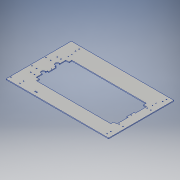
# Autodesk Inventor part: Hopper Top
Saved by Autodesk Inventor 2018 (Build 220112000, 112)
## iProperties
Created: 2013-10-16
Part Number: Hopper Top
Material: Aluminum 6061
Document SubType Name: Modeling
Designer: Gabriel Smolnycki
Mass: 1199.4 g
Surface Area: 2361.58 cm^2
Volume: 444.221 cm^3
Density: 2.7 g/cm^3
Appearance: Aluminum - Flat
Sending System: SolidWorks 2017
Last Author: Gabriel Smolnycki
Last Saved: 2017-09-14
Author: Gabriel Smolnycki
Autodesk Inventor part; units mm, degrees
ref_plane "YZ Plane" through (0, 0, 0) normal (1, 0, 0) x (0, 1, 0)
ref_plane "XY Plane" through (0, 0, 0) normal (0, 0, 1) x (1, 0, 0)
ref_plane "Work Plane1" through (0, -4, 0) normal (0, 1, 0) x (-1, 0, 0)
sketch "Sketch1" plane through (0, -4, 0) normal (0, 1, 0) x (-1, 0, 0)
  line L0 (209, 19.5) -> (209, -19.5)
  line L1 (-216.3969, -79.4609) -> (-199.5, -79.4609)
  line L2 (221, -27.5) -> (216.3969, -27.5)
  line L3 (-209, -19.5) -> (-209, 19.5)
  line L4 (290, 167.5) -> (-260, 167.5)
  line L5 (-199.5, 79.4609) -> (-216.3969, 79.4609)
  line L6 (-260, -182.5) -> (290, -182.5)
  line L7 (199.5, 79.4609) -> (199.5, 95)
  line L8 (221, 47.5) -> (216.3969, 47.5)
  line L9 (216.3969, -79.4609) -> (216.3969, -47.5)
  line L10 (216.3969, 19.5) -> (216.3969, 27.5)
  line L11 (-199.5, -95) -> (199.5, -95)
  line L12 (209, -19.5) -> (216.3969, -19.5)
  line L13 (-216.3969, -19.5) -> (-216.3969, -79.4609)
  arc A0 (221, -47.5) -> (221, -27.5) centre (221, -37.5) ccw
  line L14 (-209, 19.5) -> (-216.3969, 19.5)
  line L15 (-199.5, 95) -> (-199.5, 79.4609)
  line L16 (-260, 167.5) -> (-260, -182.5)
  line L17 (216.3969, 79.4609) -> (199.5, 79.4609)
  arc A1 (221, 27.5) -> (221, 47.5) centre (221, 37.5) ccw
  line L18 (199.5, -79.4609) -> (216.3969, -79.4609)
  line L19 (290, -182.5) -> (290, 167.5)
  line L20 (216.3969, 19.5) -> (209, 19.5)
  line L21 (-199.5, -79.4609) -> (-199.5, -95)
  line L22 (216.3969, -27.5) -> (216.3969, -19.5)
  line L23 (-216.3969, -19.5) -> (-209, -19.5)
  line L24 (216.3969, -47.5) -> (221, -47.5)
  line L25 (-216.3969, 79.4609) -> (-216.3969, 19.5)
  line L26 (199.5, 95) -> (-199.5, 95)
  line L27 (216.3969, 47.5) -> (216.3969, 79.4609)
  line L28 (216.3969, 27.5) -> (221, 27.5)
  line L29 (199.5, -95) -> (199.5, -79.4609)
  point P0 (0, 0)
  dimension "d194" = 79.4609
  dimension "d195" = 216.3969
  dimension "d196" = 216.3969
  dimension "d197" = 79.4609
  dimension "d198" = 209
  dimension "d199" = 19.5
  dimension "d201" = 20
  dimension "d202" = 27.5
  dimension "d203" = 10
  dimension "d204" = 95
  dimension "d205" = 199.5
  dimension "d206" = 260
  dimension "d207" = 550
  dimension "d208" = 182.5
  dimension "d209" = 350
  dimension "d210" = 221
  dimension "d211" = 4.6031
  constraints: 60 end point, 16 horizontal, 14 vertical, 13 equal length, 6 collinear, 4 point on circle, 2 centre point, 1 equal radius, 1 other
  measures "d194" distance from line of L18 point (0, 0)
  measures "d195" distance from line of point (0, 0) L9
  measures "d196" distance from line of L13 point (0, 0)
  measures "d197" distance from line of L17 point (0, 0)
  measures "d198" distance from line of L0 point (0, 0)
  measures "d199" distance from line of L12 point (0, 0)
  measures "d201" distance between parallel lines of L2 L24
  measures "d202" distance from line of L2 point (0, 0)
  measures "d203" radius of A0
  measures "d204" distance from line of point (0, 0) L11
  measures "d205" distance from line of point (0, 0) L29
  measures "d206" distance from line of L16 point (0, 0)
  measures "d207" distance between parallel lines of L19 L16
  measures "d208" distance from line of L6 point (0, 0)
  measures "d209" distance between parallel lines of L4 L6
  measures "d210" horizontal distance of point (0, 0) L2.start
  measures "d211" distance of L9.end L24.end
extrude "Extrusion2" add sketch "Sketch1" along normal blind 4
sketch "Sketch2" plane through (0, 0, 0) normal (0, 1, 0) x (-1, 0, 0)
  arc A0 (144, 149.75) -> (144, 145.25) centre (144, 147.5) ccw
  line L0 (154, 149.75) -> (144, 149.75)
  line L1 (144, 145.25) -> (154, 145.25)
  arc A1 (154, 145.25) -> (154, 149.75) centre (154, 147.5) ccw
  constraints: 4 end point, 4 point on circle, 2 centre point, 2 horizontal, 1 equal radius, 1 parallel
extrude "Extrusion1" cut sketch "Sketch2" against normal blind 4
hole "Hole27" at (-281.5, -4, 37.5) direction (0, 1, 0) diameter 4.5 depth 4
hole "Hole26" at (-256.5, -4, -37.5) direction (0, 1, 0) diameter 4.5 depth 4
hole "Hole25" at (-281.5, -4, -37.5) direction (0, 1, 0) diameter 4.5 depth 4
hole "Hole24" at (214, -4, 0) direction (0, 1, 0) diameter 3.5 depth 4
hole "Hole23" at (-214, -4, 0) direction (0, 1, 0) diameter 3.5 depth 4
hole "Hole22" at (-284, -4, 147.5) direction (0, 1, 0) diameter 4.5 depth 4
hole "Hole21" at (236, -4, 131.5) direction (0, 1, 0) diameter 4.5 depth 4
hole "Hole20" at (236, -4, 151.5) direction (0, 1, 0) diameter 4.5 depth 4
hole "Hole19" at (236, -4, -166.5) direction (0, 1, 0) diameter 4.5 depth 4
hole "Hole18" at (236, -4, -146.5) direction (0, 1, 0) diameter 4.5 depth 4
hole "Hole17" at (-232, -4, 131.5) direction (0, 1, 0) diameter 4.5 depth 4
hole "Hole16" at (-232, -4, 151.5) direction (0, 1, 0) diameter 4.5 depth 4
hole "Hole15" at (-232, -4, -166.5) direction (0, 1, 0) diameter 4.5 depth 4
sketch "Sketch16" plane through (0, -4, 0) normal (0, 1, 0) x (-1, 0, 0)
  point P0 (232, -146.5)
hole "Hole14" at (-232, -4, -146.5) direction (0, 1, 0) diameter 4.5 depth 4
sketch "Sketch15" plane through (0, -4, 0) normal (0, 1, 0) x (-1, 0, 0)
  point P0 (232, -166.5)
hole "Hole13" at (225.5, -4, -121) direction (0, 1, 0) diameter 3.5 depth 4
sketch "Sketch14" plane through (0, -4, 0) normal (0, 1, 0) x (-1, 0, 0)
  point P0 (232, 151.5)
hole "Hole12" at (225.5, -4, -102) direction (0, 1, 0) diameter 3.5 depth 4
sketch "Sketch13" plane through (0, -4, 0) normal (0, 1, 0) x (-1, 0, 0)
  point P0 (232, 131.5)
hole "Hole11" at (-225.5, -4, -121) direction (0, 1, 0) diameter 3.5 depth 4
sketch "Sketch12" plane through (0, -4, 0) normal (0, 1, 0) x (-1, 0, 0)
  point P0 (-236, -146.5)
hole "Hole10" at (-225.5, -4, -102) direction (0, 1, 0) diameter 3.5 depth 4
sketch "Sketch11" plane through (0, -4, 0) normal (0, 1, 0) x (-1, 0, 0)
  point P0 (-236, -166.5)
hole "Hole9" at (244, 0, -75) direction (0, -1, 0) diameter 4.5 depth 4
sketch "Sketch10" plane through (0, -4, 0) normal (0, 1, 0) x (-1, 0, 0)
  point P0 (-236, 151.5)
hole "Hole8" at (224, 0, -75) direction (0, -1, 0) diameter 4.5 depth 4
sketch "Sketch9" plane through (0, -4, 0) normal (0, 1, 0) x (-1, 0, 0)
  point P0 (-236, 131.5)
hole "Hole7" at (244, 0, 75) direction (0, -1, 0) diameter 4.5 depth 4
sketch "Sketch8" plane through (0, -4, 0) normal (0, 1, 0) x (-1, 0, 0)
  point P0 (284, 147.5)
hole "Hole6" at (224, 0, 75) direction (0, -1, 0) diameter 4.5 depth 4
sketch "Sketch7" plane through (0, -4, 0) normal (0, 1, 0) x (-1, 0, 0)
  point P0 (214, 0)
hole "Hole5" at (-256.5, -4, 37.5) direction (0, 1, 0) diameter 4.5 depth 4
sketch "Sketch6" plane through (0, -4, 0) normal (0, 1, 0) x (-1, 0, 0)
  point P0 (-214, 0)
hole "Hole4" at (-234, 0, -71) direction (0, -1, 0) diameter 4.5 depth 4
sketch "Sketch5" plane through (0, -4, 0) normal (0, 1, 0) x (-1, 0, 0)
  point P0 (281.5, -37.5)
hole "Hole3" at (-254, 0, -71) direction (0, -1, 0) diameter 4.5 depth 4
sketch "Sketch4" plane through (0, -4, 0) normal (0, 1, 0) x (-1, 0, 0)
  point P0 (256.5, -37.5)
hole "Hole2" at (-254, 0, 71) direction (0, -1, 0) diameter 4.5 depth 4
sketch "Sketch3" plane through (0, -4, 0) normal (0, 1, 0) x (-1, 0, 0)
  point P0 (281.5, 37.5)
hole "Hole1" at (-234, 0, 71) direction (0, -1, 0) diameter 4.5 depth 4
sketch "Sketch17" plane through (0, -4, 0) normal (0, 1, 0) x (-1, 0, 0)
  point P0 (-225.5, -121)
sketch "Sketch18" plane through (0, -4, 0) normal (0, 1, 0) x (-1, 0, 0)
  point P0 (-225.5, -102)
sketch "Sketch19" plane through (0, -4, 0) normal (0, 1, 0) x (-1, 0, 0)
  point P0 (225.5, -121)
sketch "Sketch20" plane through (0, -4, 0) normal (0, 1, 0) x (-1, 0, 0)
  point P0 (225.5, -102)
sketch "Sketch21" plane through (0, 0, 0) normal (0, 1, 0) x (-1, 0, 0)
  point P0 (-244, -75)
sketch "Sketch22" plane through (0, 0, 0) normal (0, 1, 0) x (-1, 0, 0)
  point P0 (-224, -75)
sketch "Sketch23" plane through (0, 0, 0) normal (0, 1, 0) x (-1, 0, 0)
  point P0 (-244, 75)
sketch "Sketch24" plane through (0, 0, 0) normal (0, 1, 0) x (-1, 0, 0)
  point P0 (-224, 75)
sketch "Sketch25" plane through (0, -4, 0) normal (0, 1, 0) x (-1, 0, 0)
  point P0 (256.5, 37.5)
sketch "Sketch26" plane through (0, 0, 0) normal (0, 1, 0) x (-1, 0, 0)
  point P0 (234, -71)
sketch "Sketch27" plane through (0, 0, 0) normal (0, 1, 0) x (-1, 0, 0)
  point P0 (254, -71)
sketch "Sketch28" plane through (0, 0, 0) normal (0, 1, 0) x (-1, 0, 0)
  point P0 (254, 71)
sketch "Sketch29" plane through (0, 0, 0) normal (0, 1, 0) x (-1, 0, 0)
  point P0 (234, 71)
equation "\"d197\" = d194"
body "Solid3"
